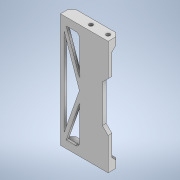
# Autodesk Inventor part: structural-bar
Saved by Autodesk Inventor 2021 (Build 250183000, 183)
## iProperties
Created: 2024-04-27
Part Number: structural-bar
Material: Generic
Document SubType Name: Modeling
Designer: Toby
Density: 1 g/cm^3
Appearance: Default
Author: Toby
Autodesk Inventor part; units mm, degrees
ref_plane "YZ Plane" through (0, 0, 0) normal (1, 0, 0) x (0, 1, 0)
ref_plane "XZ Plane" through (0, 0, 0) normal (0, 1, 0) x (-1, 0, 0)
ref_plane "XY Plane" through (0, 0, 0) normal (0, 0, 1) x (1, 0, 0)
sketch "Sketch1" plane through (0, 0, 0) normal (0, 0, 1) x (1, 0, 0)
  line L0 (-11.1895, 18.0847) -> (3.8105, 18.0847)
  line L1 (3.8105, 18.0847) -> (3.8105, -41.9153)
  line L2 (3.8105, -41.9153) -> (-11.1895, -41.9153)
  line L3 (-11.1895, -41.9153) -> (-11.1895, 18.0847)
  point P0 (0, 0)
  dimension "d0" = 15
  dimension "d1" = 60
  constraints: 8 end point, 2 parallel, 1 horizontal, 1 perpendicular
  measures "d0" distance of L0.start L0.end
  measures "d1" distance of L0.end L1.end
extrude "Extrusion1" add sketch "Sketch1" along normal blind 2
sketch "Sketch2" plane through (-11.1895, -41.9153, 0) normal (0, -1, 0) x (1, 0, 0)
  line L0 (0, 2) -> (15, 2) projected
  line L1 (0, 2) -> (15, 2)
  line L2 (15, 2) -> (15, -4)
  line L3 (15, -4) -> (0, -4)
  line L4 (0, -4) -> (0, 2)
  line L5 (15, 0) -> (15, 2) projected
  point P0 (11.1895, 0)
  dimension "d4" = 6
  constraints: 8 end point, 2 parallel, 1 collinear, 1 horizontal, 1 perpendicular
  measures "d4" distance between parallel lines of L3 L0
extrude "Extrusion2" add sketch "Sketch2" against normal blind 3
sketch "Sketch3" plane through (-11.1895, 18.0847, 0) normal (0, 1, 0) x (1, 0, 0)
  line L0 (0, -2) -> (15, -2) projected
  line L1 (0, -2) -> (0, 4) projected
  line L2 (15, -2) -> (0, -2)
  line L3 (0, -2) -> (0, 4)
  line L4 (0, 4) -> (15, 4)
  line L5 (15, 4) -> (15, -2)
  point P0 (11.1895, 0)
  constraints: 8 end point, 2 parallel, 1 horizontal, 1 perpendicular
extrude "Extrusion3" add sketch "Sketch3" against normal blind 3
chamfer "Chamfer1" distance 3 angle 45 2 edges at (-3.6895, 15.0847, 0) (-3.6895, -38.9153, 0)
sketch "Sketch4" plane through (-11.1895, -41.9153, 2) normal (0, -1, 0) x (1, 0, 0)
  line L0 (15, -6) -> (15, 0) projected
  line L1 (0, 0) -> (15, 0) projected
  point P0 (11.1895, -2)
  point P1 (12, -3)
  point P2 (3, -3)
  dimension "d12" = 3
  dimension "d13" = 12
  dimension "d14" = 3
  dimension "d15" = 3
  measures "d12" distance from line of L0 point (12, -3)
  measures "d13" distance from line of L0 point (3, -3)
  measures "d14" distance from line of L1 point (12, -3)
  measures "d15" distance from line of L1 point (3, -3)
hole "Hole1" at (0.8105, -41.9153, -1) at (-8.1895, -41.9153, -1) direction (0, 1, 0) diameter 2 depth 3 tip angle 118
sketch "Sketch5" plane through (-11.1895, 18.0847, 2) normal (0, 1, 0) x (1, 0, 0)
  circle A0 centre (12, 3) radius 1 projected
  circle A1 centre (3, 3) radius 1 projected
  point P0 (11.1895, 2)
  constraints: 2 coincident
hole "Hole2" at (0.8105, 18.0847, -1) at (-8.1895, 18.0847, -1) direction (0, -1, 0) diameter 2 depth 3 tip angle 118
sketch "Sketch6" plane through (0, 0, 2) normal (0, 0, 1) x (1, 0, 0)
  line L0 (3.8105, -41.9153) -> (-11.1895, -41.9153)
  line L1 (-11.1895, -41.9153) -> (-11.1895, -41.8153)
  line L2 (-11.1895, -41.8153) -> (3.8105, -41.8153)
  line L3 (3.8105, -41.8153) -> (3.8105, -41.9153)
  line L4 (3.8105, 17.9847) -> (-11.1895, 17.9847)
  line L5 (-11.1895, 17.9847) -> (-11.1895, 18.0847)
  line L6 (-11.1895, 18.0847) -> (3.8105, 18.0847)
  line L7 (3.8105, 18.0847) -> (3.8105, 17.9847)
  line L8 (3.8105, -41.9153) -> (3.8105, 18.0847) projected
  line L9 (3.8105, 18.0847) -> (-11.1895, 18.0847) projected
  line L10 (-11.1895, 18.0847) -> (-11.1895, -41.9153) projected
  line L11 (-11.1895, -41.9153) -> (3.8105, -41.9153) projected
  point P0 (0, 0)
  dimension "d30" = 0.1
  dimension "d31" = 0.1
  constraints: 16 end point, 5 collinear, 4 parallel, 2 horizontal, 2 perpendicular, 1 point on line
  measures "d30" distance between parallel lines of L0 L2
  measures "d31" distance between parallel lines of L6 L4
extrude "Extrusion4" cut sketch "Sketch6" against normal blind 30 contours L0 L1 L2 L3 | L4 L5 L6 L7
chamfer "Chamfer2" distance 2 angle 45 2 edges at (3.8105, -40.3653, -4) (3.8105, 16.5347, -4)
chamfer "Chamfer3" distance 2 angle 45 2 edges at (-11.1895, 16.5347, -4) (-11.1895, -40.3653, -4)
sketch "Sketch7" plane through (0, 0, 2) normal (0, 0, 1) x (1, 0, 0)
  line L0 (3.8105, -41.8153) -> (3.8105, 17.9847) projected
  line L1 (3.8105, -2.0153) -> (0.8105, -2.0153)
  line L2 (0.8105, -2.0153) -> (0.8105, -21.8153)
  line L3 (0.8105, -21.8153) -> (3.8105, -21.8153)
  line L4 (3.8105, -21.8153) -> (3.8105, -2.0153)
  line L5 (3.8105, 17.9847) -> (-11.1895, 17.9847) projected
  line L6 (-11.1895, -41.8153) -> (3.8105, -41.8153) projected
  point P0 (0, 0)
  dimension "d40" = 3
  dimension "d41" = 20
  dimension "d42" = 20
  constraints: 8 end point, 2 parallel, 1 horizontal, 1 perpendicular, 1 point on line
  measures "d40" distance between parallel lines of L0 L2
  measures "d41" distance between parallel lines of L5 L1
  measures "d42" distance between parallel lines of L6 L3
extrude "Extrusion5" cut sketch "Sketch7" against normal blind 2
chamfer "Chamfer4" distance 3 angle 45 2 edges at (3.8105, -2.0153, 1) (3.8105, -21.8153, 1)
sketch "Sketch8" plane through (0, 0, 2) normal (0, 0, 1) x (1, 0, 0)
  line L0 (-11.1895, 14.0847) -> (-11.1895, 17.9847) projected
  line L1 (-11.1895, 17.9847) -> (-21.1895, 17.9847)
  line L2 (-21.1895, 17.9847) -> (-21.1895, -41.8153)
  line L3 (-21.1895, -41.8153) -> (-11.1895, -41.8153)
  line L4 (-11.1895, -41.8153) -> (-11.1895, 17.9847)
  line L5 (-11.1895, -41.8153) -> (3.8105, -41.8153) projected
  point P0 (0, 0)
  dimension "d48" = 10
  constraints: 8 end point, 2 parallel, 1 collinear, 1 horizontal, 1 perpendicular
  measures "d48" distance between parallel lines of L4 L2
extrude "Extrusion6" add sketch "Sketch8" against normal blind 1.2
chamfer "Chamfer5" distance 0.8 angle 45 1 edges at (-11.1895, -11.9153, 0)
sketch "Sketch9" plane through (0, 0, 0.8) normal (0, 0, -1) x (-1, 0, 0)
  line L0 (9.1895, 15.0847) -> (9.1895, 17.9847) projected
  line L1 (21.1895, 17.9847) -> (21.1895, -41.8153) projected
  line L2 (9.1895, 17.9847) -> (21.1895, 17.9847)
  line L3 (21.1895, 17.9847) -> (21.1895, 15.9847)
  line L4 (21.1895, 15.9847) -> (9.1895, 15.9847)
  line L5 (9.1895, 15.9847) -> (9.1895, 17.9847)
  line L6 (9.1895, -38.9153) -> (9.1895, -41.8153) projected
  line L7 (9.1895, -41.8153) -> (21.1895, -41.8153)
  line L8 (21.1895, -41.8153) -> (21.1895, -39.8153)
  line L9 (21.1895, -39.8153) -> (9.1895, -39.8153)
  line L10 (9.1895, -39.8153) -> (9.1895, -41.8153)
  line L11 (21.1895, 17.9847) -> (11.1895, 17.9847) projected
  point P0 (0, 0)
  point P1 (21.1895, -39.8153)
  point P2 (9.1895, -39.8153)
  point P3 (9.1895, 15.9847)
  dimension "d54" = 2
  dimension "d55" = 2
  constraints: 16 end point, 4 parallel, 3 point on line, 2 horizontal, 2 perpendicular, 1 collinear
  measures "d54" distance between parallel lines of L7 L9
  measures "d55" distance between parallel lines of L2 L4
extrude "Extrusion7" add sketch "Sketch9" along normal blind 4.8
chamfer "Chamfer6" distance 2 angle 45 2 edges at (-21.1895, -40.8153, -4) (-21.1895, 16.9847, -4)
sketch "Sketch10" plane through (0, 0, 0.8) normal (0, 0, -1) x (-1, 0, 0)
  line L0 (11.1895, -39.8153) -> (11.1895, -35.1153) projected
  line L1 (11.1895, -37.8153) -> (19.1895, -37.8153)
  line L2 (19.1895, -37.8153) -> (19.1895, 13.9847)
  line L3 (19.1895, 13.9847) -> (11.1895, 13.9847)
  line L4 (11.1895, 13.9847) -> (11.1895, -37.8153)
  line L5 (9.1895, 15.9847) -> (19.1895, 15.9847) projected
  line L6 (21.1895, -39.8153) -> (21.1895, 15.9847) projected
  line L7 (19.1895, -39.8153) -> (9.1895, -39.8153) projected
  point P0 (0, 0)
  dimension "d61" = 2
  dimension "d62" = 2
  dimension "d63" = 2
  constraints: 8 end point, 2 parallel, 1 horizontal, 1 perpendicular, 1 point on line
  measures "d61" distance between parallel lines of L3 L5
  measures "d62" distance between parallel lines of L6 L2
  measures "d63" distance between parallel lines of L7 L1
extrude "Extrusion8" cut sketch "Sketch10" against normal blind 2
fillet "Fillet1" radius 2 2 edges at (-11.1895, 13.9847, 1.4) (-11.1895, -37.8153, 1.4)
sketch "Sketch12" plane through (0, 0, 2) normal (0, 0, 1) x (1, 0, 0)
  line L0 (-11.1895, -35.1153) -> (-11.1895, 11.2847) projected
  line L1 (-19.1895, 13.9847) -> (-13.1895, 13.9847) projected
  line L2 (-13.1895, -37.8153) -> (-19.1895, -37.8153) projected
  line L3 (-19.1895, -37.8153) -> (-19.1895, 13.9847) projected
  line L4 (-19.1895, -37.8153) -> (-10.1895, -11.9153) construction
  line L5 (-18.2449, -38.1436) -> (-9.2449, -12.2436)
  line L6 (-11.1341, -11.5871) -> (-20.1341, -37.4871)
  arc A0 (-20.1341, -37.4871) -> (-18.2449, -38.1436) centre (-19.1895, -37.8153) ccw
  arc A1 (-9.2449, -12.2436) -> (-11.1341, -11.5871) centre (-10.1895, -11.9153) ccw
  line L7 (-10.1895, -11.9153) -> (-19.1895, 13.9847) construction
  line L8 (-9.2449, -11.5871) -> (-18.2449, 14.3129)
  line L9 (-20.1341, 13.6564) -> (-11.1341, -12.2436)
  arc A2 (-11.1341, -12.2436) -> (-9.2449, -11.5871) centre (-10.1895, -11.9153) ccw
  arc A3 (-18.2449, 14.3129) -> (-20.1341, 13.6564) centre (-19.1895, 13.9847) ccw
  point P0 (0, 0)
  point P1 (-11.1895, -11.9153)
  point P2 (-14.6895, -24.8653)
  point P3 (-14.6895, 1.0347)
  point P4 (-19.1895, 10.9381)
  point P5 (-11.2482, -11.9153)
  point P6 (-19.1895, -34.7688)
  point P7 (-18.1309, -37.8153)
  point P8 (-11.1895, -17.8397)
  point P9 (-11.1895, -5.991)
  point P10 (-18.1309, 13.9847)
  dimension "d71" = 1
  dimension "d72" = 51.8
  dimension "d73" = 25.9
  dimension "d74" = 2
  dimension "d75" = 2
  constraints: 16 end point, 8 point on circle, 8 tangent, 4 centre point, 3 midpoint, 2 parallel
  measures "d71" distance of L4.end point (-11.19, -11.915)
  measures "d72" distance between parallel lines of L1 L2
  measures "d73" distance from line of L4.end L2
  measures "d74" diameter of A1
  measures "d75" diameter of A3
extrude "Extrusion10" add sketch "Sketch12" against normal blind 1.2 contours L5 L2 L3 L6 L9 L0 | L9 L6 L0 | L6 L9 L3 L1 L8 L0
body "Solid1"
